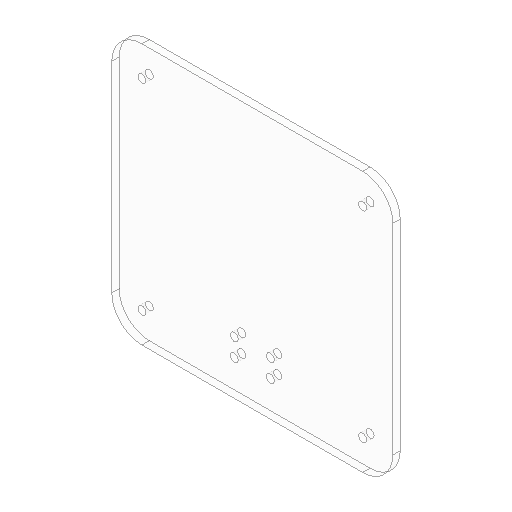
# Autodesk Inventor part: Base
Saved by Autodesk Inventor 2025.3 (Build 293356000, 356)
## iProperties
Created: 2025-11-11
Part Number: Base
Material: Polycarbonate, Clear
Document SubType Name: Modeling
Designer: Gabriel Bojaca
Density: 1.2 g/cm^3
Appearance: Polycarbonate - Clear
Author: Gabriel Bojaca
Autodesk Inventor part; units mm, degrees
ref_plane "YZ Plane" through (0, 0, 0) normal (1, 0, 0) x (0, 1, 0)
ref_plane "XZ Plane" through (0, 0, 0) normal (0, 1, 0) x (-1, 0, 0)
ref_plane "XY Plane" through (0, 0, 0) normal (0, 0, 1) x (1, 0, 0)
sketch "Sketch1" plane through (0, 0, 0) normal (0, 0, 1) x (1, 0, 0)
  line L0 (15, 0) -> (125, 0)
  line L1 (140, 15) -> (140, 115)
  line L2 (125, 130) -> (15, 130)
  line L3 (0, 115) -> (0, 15)
  arc A0 (15, 130) -> (0, 115) centre (15, 115) ccw
  arc A1 (140, 115) -> (125, 130) centre (125, 115) ccw
  arc A2 (125, 0) -> (140, 15) centre (125, 15) ccw
  arc A3 (0, 15) -> (15, 0) centre (15, 15) ccw
  circle A4 centre (15, 115) radius 2
  circle A5 centre (125, 115) radius 2
  circle A6 centre (15, 15) radius 2
  circle A7 centre (125, 15) radius 2
  line L4 (61, 17.5) -> (79, 17.5) construction
  line L5 (79, 17.5) -> (79, 26.5) construction
  line L6 (79, 26.5) -> (61, 26.5) construction
  line L7 (61, 26.5) -> (61, 17.5) construction
  line L8 (61, 17.5) -> (79, 26.5) construction
  line L9 (79, 17.5) -> (61, 26.5) construction
  line L10 (70, 0) -> (70, 130) construction
  circle A8 centre (61, 26.5) radius 2
  circle A9 centre (61, 17.5) radius 2
  circle A10 centre (79, 26.5) radius 2
  circle A11 centre (79, 17.5) radius 2
  point P0 (0, 0)
  point P1 (140, 130)
  point P2 (140, 0)
  point P3 (0, 130)
  point P4 (70, 22)
  point P5 (70, 17.5)
  dimension "d0" = 140
  dimension "d1" = 130
  dimension "d2" = 15
  dimension "d3" = 4
  dimension "d4" = 4
  dimension "d5" = 4
  dimension "d6" = 4
  dimension "d7" = 18
  dimension "d8" = 9
  dimension "d9" = 17.5
  dimension "d11" = 4
  dimension "d12" = 4
  constraints: 22 end point, 12 centre point, 9 point on line, 8 point on circle, 8 tangent, 6 coincident, 5 midpoint, 4 parallel, 3 equal radius, 2 horizontal, 2 perpendicular, 2 symmetric about line, 2 other
  measures "d0" distance of point (0, 130) point (140, 130)
  measures "d1" distance of point (140, 130) point (140, 0)
  measures "d2" radius of A0
  measures "d3" diameter of A4
  measures "d4" diameter of A5
  measures "d5" diameter of A6
  measures "d6" diameter of A7
  measures "d7" distance of L6.end L5.end
  measures "d8" distance of L5.end L4.end
  measures "d9" distance from line of L0 point (70, 17.5)
  measures "d11" diameter of A8
  measures "d12" diameter of A9
extrude "Extrusion1" add sketch "Sketch1" along normal blind 3.7
body "Solid1"
